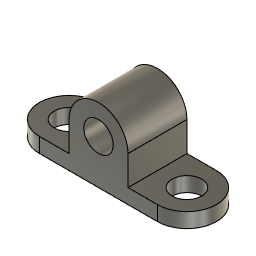
A4 (Autodesk Fusion 360 design; units mm, degrees)
Autodesk Fusion 360 part; units mm, degrees
note: some values were not read from the file. Set by a fixed rule: the direction of a hole.
sketch "Sketch1" plane through (0, 0, 0) normal (0, 0, 1) x (1, 0, 0)
  line L0 (40, 20) -> (-40, 20)
  line L1 (-40, 20) -> (-40, -20)
  line L2 (-40, -20) -> (40, -20)
  line L3 (40, -20) -> (40, 20)
  line L4 (40, 20) -> (-40, -20) construction
  line L5 (-40, 20) -> (40, -20) construction
  line L6 (-40, -20) -> (-20, -20) construction
  line L7 (-40, -20) -> (-20, -20) construction
  line L8 (40, -20) -> (20, -20) construction
  line L9 (-20, -20) -> (-20, 20)
  line L10 (20, -20) -> (20, 20)
  line L11 (-40, -20) -> (-60, -20)
  line L12 (-40, 20) -> (-60, 20)
  line L13 (-60, 20) -> (-60, -20)
  line L14 (40, 20) -> (60, 20)
  line L15 (60, 20) -> (60, -20)
  line L16 (60, -20) -> (40, -20)
  line L17 (-40, 0) -> (-40, 20) construction
  line L18 (40, 20) -> (40, 0) construction
  dimension "d1" = 80
  dimension "d2" = 40
  dimension "d3" = 20
  dimension "d4" = 20
  dimension "d5" = 20
  constraint horizontal L0
  constraint perpendicular L0 L1
  constraint parallel L0 L2
  constraint parallel L1 L3
  constraint coincident L4 origin
  constraint coincident L5 origin
  constraint coincident L2 L6.end
  constraint coincident L2 L8.end
  constraint coincident L0 L9.end
  constraint perpendicular L0 L9
  constraint coincident L0 L10.end
  constraint perpendicular L0 L10
  constraint perpendicular L1 L11
  constraint perpendicular L1 L12
  constraint perpendicular L11 L13
  constraint perpendicular L3 L14
  constraint perpendicular L14 L15
  constraint perpendicular L3 L16
  constraint midpoint L1 L17.start
  constraint midpoint L3 L18.end
  measures "d1" distance of L1.end L2.end
  measures "d2" distance of L0.end L1.end
  measures "d3" distance of L1.end L6.end
  measures "d4" distance of L2.end L8.end
  measures "d5" distance of L1.end L11.end
extrude "Extrude2" add sketch "Sketch1" along normal blind 50 contours L0 L2 L9 L10 makes body 1
extrude "Extrude1" add sketch "Sketch1" along normal blind 10 separate body contours L0 L2 L3 L10 | L3 L14 L15 L16 | L0 L1 L2 L9 | L1 L11 L12 L13 makes body 2 at (-33.3333, -6.6667, 0) makes body 3 at (46.6667, -6.6667, 0)
fillet "Fillet1" radius 20 4 edges at (-60, -20, 5) (-60, 20, 5) (60, -20, 5) (60, 20, 5) on bodies 2 3
hole "Hole1" at (-40, 0, 0) direction (0, 0, 1) diameter 20 depth 10 tip angle 118 bodies 2
hole "Hole2" at (40, 0, 0) direction (0, 0, 1) diameter 20 depth 10 tip angle 118 bodies 3
fillet "Fillet2" radius 20 2 edges at (-20, 0, 50) (20, 0, 50) on bodies 1
sketch "Sketch2" plane through (0, -20, 0) normal (0, -1, 0) x (1, 0, 0)
  arc A0 (20, 30) -> (-20, 30) centre (0, 30) ccw
  line L0 (-20, 30) -> (-20, 0)
  line L1 (-20, 0) -> (20, 0)
  line L2 (20, 0) -> (20, 30)
  line L3 (-20, 30) -> (20, 30) construction
  constraint coincident A0.end L0.start
  constraint coincident A0.start L2.end
hole "Hole3" at (0, -20, 30) direction (0, 1, 0) diameter 20 depth 40 tip angle 118 bodies 1
combine "Combine1" operation add target body 2 tool bodies 3 1
